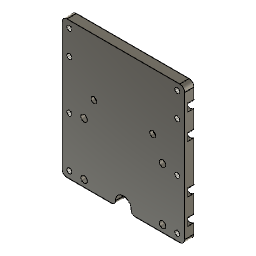
JRCNC0010 v28 (Autodesk Fusion 360 design; units mm, degrees)
Autodesk Fusion 360 part; units mm, degrees
sketch "Sketch1" plane through (0, 0, 0) normal (0, 1, 0) x (1, 0, 0)
  line L0 (22.5, -7) -> (22.5, -61) construction
  line L1 (121, -45) -> (121, -19) construction
  line L2 (95, -120) -> (121, -120) construction
  line L3 (22.5, -61) -> (102.5, -61) construction
  line L4 (102.5, -61) -> (102.5, -7) construction
  line L5 (95, -94) -> (95, -120) construction
  line L6 (30, -19) -> (4, -19) construction
  line L7 (121, -19) -> (95, -19) construction
  line L8 (32.5, -82) -> (92.5, -82) construction
  line L9 (125, 0) -> (74.4896, 0)
  line L10 (4, -45) -> (30, -45) construction
  arc A0 (54.5069, -4.1667) -> (70.4931, -4.1667) centre (62.5, -4.5) ccw
  line L11 (50.5104, 0) -> (0, 0)
  line L12 (4, -120) -> (30, -120) construction
  line L13 (30, -94) -> (4, -94) construction
  line L14 (102.5, -7) -> (22.5, -7) construction
  arc A1 (74.4896, 0) -> (70.4931, -4.1667) centre (74.4896, -4) ccw
  arc A2 (54.5069, -4.1667) -> (50.5104, 0) centre (50.5104, -4) ccw
  line L15 (30, -120) -> (30, -94) construction
  line L16 (95, -45) -> (121, -45) construction
  line L17 (125, -140) -> (125, 0)
  line L18 (4, -94) -> (4, -120) construction
  line L19 (95, -19) -> (95, -45) construction
  line L20 (121, -94) -> (95, -94) construction
  line L21 (4, -19) -> (4, -45) construction
  line L22 (121, -120) -> (121, -94) construction
  line L23 (30, -45) -> (30, -19) construction
  line L24 (0, -140) -> (125, -140)
  line L25 (62.5, -140) -> (62.5, 80) construction
  line L26 (0, 0) -> (0, -140)
  dimension "d19" = 26
  dimension "d20" = 26
  dimension "d21" = 26
  dimension "d22" = 20
  dimension "d23" = 140
  dimension "d55" = 40
  dimension "d56" = 40
  dimension "d28" = 49
  dimension "d29" = 54
  dimension "d34" = 82
  dimension "d36" = 16
  dimension "d37" = 4.5
  dimension "d39" = 8
  dimension "d44" = 125
  dimension "d45" = 65
  dimension "d46" = 32.5
  dimension "d47" = 60
  dimension "d50" = 30
  dimension "d51" = 7
  constraint horizontal L24
  constraint vertical L17
  constraint horizontal L9
  constraint vertical L26
  constraint horizontal L10
  constraint vertical L23
  constraint horizontal L6
  constraint vertical L21
  constraint horizontal L16
  constraint vertical L1
  constraint horizontal L7
  constraint vertical L19
  constraint horizontal L12
  constraint vertical L15
  constraint horizontal L13
  constraint vertical L18
  constraint horizontal L2
  constraint vertical L22
  constraint horizontal L20
  constraint vertical L5
  constraint horizontal L3
  constraint vertical L4
  constraint horizontal L14
  constraint vertical L0
  constraint midpoint L25.start L24
  constraint perpendicular L9 L25
  constraint collinear L15 L23
  constraint collinear L5 L19
  constraint equal L18 L21
  constraint equal L5 L19
  constraint collinear L10 L16
  constraint collinear L2 L12
  constraint equal L2 L12
  constraint equal L16 L20
  constraint coincident A0.centre L25
  constraint equal L10 L13
  constraint perpendicular L8 L25
  constraint tangent L9 A2
  constraint tangent L9 A1
  constraint tangent A0 A2
  constraint tangent A0 A1
  constraint equal A1 A2
  constraint coincident L11.start L9
  constraint collinear L9 L11
  constraint coincident L11.end L26.start
  measures "d19" distance of L12.start L12.end
  measures "d20" distance of L13.start L12.end
  measures "d21" distance of L1.end L1.start
  measures "d22" distance of L12 L24
  measures "d23" distance of L11.end L24.start
  measures "d55" distance of L0.end L25
  measures "d56" distance of L4 L25
  measures "d28" distance of L10 L13
  measures "d29" distance of L4.end L3
  measures "d34" distance of L8 L9
  measures "d36" diameter of A0
  measures "d37" distance of A0.centre L9
  measures "d39" diameter of A2
  measures "d44" distance of L17.start L24.start
  measures "d45" distance of L5 L15
  measures "d46" distance of L5 L25
  measures "d47" distance of L8.end L8.start
  measures "d50" distance of L8.start L25
  measures "d51" distance of L11 L14
extrude "Extrude1" add sketch "Sketch1" against normal blind 9.525
hole "Hole2" at (95, 0, 120) at (121, 0, 120) at (121, 0, 94) at (95, 0, 94) at (30, 0, 120) at (30, 0, 94) at (4, 0, 94) at (4, 0, 120) at (121, 0, 45) at (121, 0, 19) at (95, 0, 45) at (30, 0, 45) at (4, 0, 45) at (4, 0, 19) direction (0, -1, 0) diameter 11 depth 6.1 tip angle 180
hole "Hole3" at (92.5, 0, 82) at (32.5, 0, 82) direction (0, -1, 0) diameter 6 depth 10 tip angle 180 counterbore diameter 11 counterbore depth 6.1
fillet "Fillet1" radius 5 4 edges at (125, -4.7625, 140) (125, -4.7625, 0) (0, -4.7625, 0) (0, -4.7625, 140)
sketch "Sketch4" plane through (0, 0, 0) normal (0, 1, 0) x (1, 0, 0)
  arc A0 (0, -135) -> (5, -140) centre (5, -135) ccw construction
  line L0 (0, -5) -> (0, -15.2251) construction
  arc A1 (5, 0) -> (0, -5) centre (5, -5) ccw construction
  line L1 (50.5104, 0) -> (5, 0) construction
  arc A2 (54.5069, -4.1667) -> (50.5104, 0) centre (50.5104, -4) ccw construction
  arc A3 (54.5069, -4.1667) -> (70.4931, -4.1667) centre (62.5, -4.5) ccw construction
  arc A4 (74.4896, 0) -> (70.4931, -4.1667) centre (74.4896, -4) ccw construction
  line L2 (120, 0) -> (74.4896, 0) construction
  arc A5 (125, -5) -> (120, 0) centre (120, -5) ccw construction
  line L3 (125, -135) -> (125, -123.7749) construction
  arc A6 (120, -140) -> (125, -135) centre (120, -135) ccw construction
  line L4 (5, -140) -> (120, -140) construction
  line L5 (7.5, -108) -> (117.5, -108) construction
  line L6 (117.5, -108) -> (117.5, -58) construction
  line L7 (117.5, -58) -> (7.5, -58) construction
  line L8 (7.5, -58) -> (7.5, -108) construction
  line L9 (62.5, -140) -> (62.5, -12.5) construction
  circle A7 centre (92.5, -82) radius 5.5
  circle A8 centre (32.5, -82) radius 5.5
  arc A9 (125, -116.2251) -> (125, -123.7749) centre (121, -120) ccw
  line L10 (125, -116.2251) -> (125, -97.7749)
  arc A10 (125, -90.2251) -> (125, -97.7749) centre (121, -94) ccw
  line L11 (125, -90.2251) -> (125, -48.7749)
  arc A11 (125, -41.2251) -> (125, -48.7749) centre (121, -45) ccw
  line L12 (125, -41.2251) -> (125, -22.7749)
  arc A12 (125, -15.2251) -> (125, -22.7749) centre (121, -19) ccw
  line L13 (125, -15.2251) -> (125, -5)
  arc A13 (0, -22.7749) -> (0, -15.2251) centre (4, -19) ccw
  line L14 (0, -22.7749) -> (0, -41.2251)
  arc A14 (0, -48.7749) -> (0, -41.2251) centre (4, -45) ccw
  line L15 (0, -48.7749) -> (0, -90.2251)
  arc A15 (0, -97.7749) -> (0, -90.2251) centre (4, -94) ccw
  line L16 (0, -97.7749) -> (0, -116.2251)
  arc A16 (0, -123.7749) -> (0, -116.2251) centre (4, -120) ccw
  line L17 (0, -123.7749) -> (0, -135)
  circle A17 centre (30, -45) radius 5.5
  circle A18 centre (30, -94) radius 5.5
  circle A19 centre (95, -94) radius 5.5
  circle A20 centre (95, -120) radius 5.5
  circle A21 centre (30, -120) radius 5.5
  circle A22 centre (95, -45) radius 5.5
  dimension "d73" = 110
  dimension "d74" = 55
  dimension "d76" = 32
  dimension "d90" = 50
  constraint horizontal L5
  constraint vertical L6
  constraint horizontal L7
  constraint vertical L8
  constraint midpoint L4 L9.start
  constraint midpoint A3 L9.end
  measures "d73" distance of L5.start L5.end
  measures "d74" distance of L6 L9
  measures "d76" distance of L4 L5
  measures "d90" distance of L5.end L6.end
hole "Hole1" at (7.5, 0, 108) at (7.5, 0, 58) at (117.5, 0, 108) at (117.5, 0, 58) direction (0, -1, 0) diameter 5.035 depth 10 tip angle 180
thread "Thread1" "ISO Metric profile 6.0 M6x1 6H"
hole "Hole4" at (102.5, 0, 61) at (22.5, 0, 61) at (22.5, 0, 7) at (102.5, 0, 7) direction (0, -1, 0) diameter 6.6 depth 10 tip angle 180
sketch "Sketch5" plane through (0, -9.525, 0) normal (0, -1, 0) x (1, 0, 0)
  circle A0 centre (22.5, 7) radius 3.3
  circle A1 centre (102.5, 61) radius 3.3
  circle A2 centre (22.5, 61) radius 3.3
  circle A3 centre (102.5, 7) radius 3.3
  circle A4 centre (117.5, 108) radius 2.5175
  circle A5 centre (7.5, 108) radius 2.5175
  circle A6 centre (7.5, 58) radius 2.5175
  circle A7 centre (117.5, 58) radius 2.5175
  arc A8 (5, 140) -> (0, 135) centre (5, 135) ccw
  line L0 (0, 135) -> (0, 5)
  arc A9 (0, 5) -> (5, 0) centre (5, 5) ccw
  line L1 (5, 0) -> (50.5104, 0)
  arc A10 (50.5104, 0) -> (54.5069, 4.1667) centre (50.5104, 4) ccw
  arc A11 (70.4931, 4.1667) -> (54.5069, 4.1667) centre (62.5, 4.5) ccw
  arc A12 (70.4931, 4.1667) -> (74.4896, 0) centre (74.4896, 4) ccw
  line L2 (74.4896, 0) -> (120, 0)
  arc A13 (120, 0) -> (125, 5) centre (120, 5) ccw
  line L3 (125, 5) -> (125, 135)
  arc A14 (125, 135) -> (120, 140) centre (120, 135) ccw
  line L4 (120, 140) -> (5, 140)
  circle A15 centre (92.5, 82) radius 3
  circle A16 centre (32.5, 82) radius 3
  line L5 (0, 133) -> (125, 133) construction
  line L6 (62.5, 140) -> (62.5, 75.63) construction
  line L7 (7.5, 133) -> (117.5, 133)
  line L8 (117.5, 133) -> (117.5, 7)
  line L9 (117.5, 7) -> (7.5, 7)
  line L10 (7.5, 7) -> (7.5, 133)
  line L11 (7.5, 133) -> (117.5, 7) construction
  line L12 (117.5, 133) -> (7.5, 7) construction
  point P0 (7.5, 133)
  point P1 (117.5, 133)
  point P2 (62.5, 70)
  dimension "d94" = 55
  dimension "d95" = 110
  dimension "d96" = 7
  dimension "d100" = 7
  constraint coincident L0 L5.start
  constraint coincident L3 L5.end
  constraint perpendicular L3 L5
  constraint midpoint L4 L6.start
  constraint perpendicular L4 L6
  constraint coincident L5 P0
  constraint coincident L5 P1
  constraint horizontal L7
  constraint perpendicular L7 L8
  constraint parallel L7 L9
  constraint parallel L8 L10
  constraint coincident P0 L7.start
  constraint coincident L11 P2
  constraint coincident L12 P2
  constraint coincident L6 P2
  measures "d94" distance of L6 P0
  measures "d95" distance of P0 P1
  measures "d96" distance of L4 L5
  measures "d100" distance of L1 L9
hole "Hole5" at (7.5, -9.525, 133) at (117.5, -9.525, 133) at (117.5, -9.525, 7) at (7.5, -9.525, 7) direction (0, 1, 0) diameter 5.035 depth 35 tip angle 118
thread "Thread2" "ISO Metric profile 6.0 M6x1 6H"
